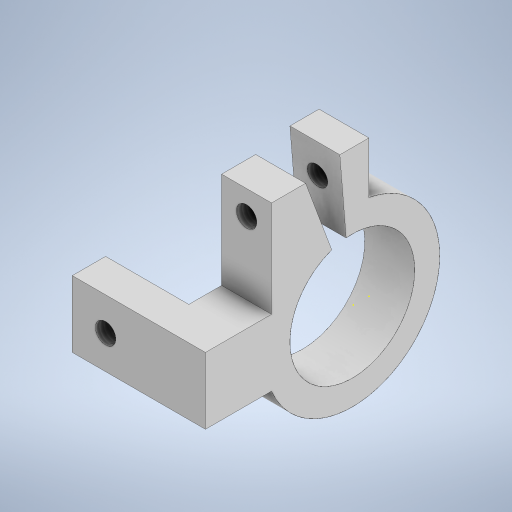
# Autodesk Inventor part: lensmount15mm
Saved by Autodesk Inventor 2023 (Build 270158000, 158)
## iProperties
Created: 2022-06-27
Part Number: lensmount15mm
Material: Generisch
Document SubType Name: Modeling
Designer: Tim Stechel
Density: 1 g/cm^3
Appearance: Vorgabe
Author: Tim Stechel
Autodesk Inventor part; units mm, degrees
ref_plane "YZ Plane" through (0, 0, 0) normal (1, 0, 0) x (0, 1, 0)
ref_plane "XZ Plane" through (0, 0, 0) normal (0, 1, 0) x (-1, 0, 0)
ref_plane "XY Plane" through (0, 0, 0) normal (0, 0, 1) x (1, 0, 0)
sketch "Skizze3" plane through (0, 0, 0) normal (0, 0, 1) x (1, 0, 0)
  line L0 (0, 0) -> (-6, 0)
  line L1 (-6, 0) -> (0, 0)
  line L2 (0, 7.5) -> (0, 10.5)
  line L3 (0, 10.5) -> (-6, 10.5)
  line L4 (-6, 10.5) -> (-6, 7.5)
  line L5 (-6, 7.5) -> (0, 7.5)
  dimension "d10" = 6
  dimension "d11" = 7.5
  dimension "d12" = 3
  dimension "d13" = 6
  constraints: 12 end point, 3 perpendicular, 1 collinear, 1 horizontal
  measures "d10" distance of L0.start L0.end
  measures "d11" distance of L0.start L2.start
  measures "d12" distance of L2.start L2.end
  measures "d13" distance of L2.end L3.end
revolve "Umdrehung2" add sketch "Skizze3" angle 335 about axis through (0, 0, 0) along (-1, 0, 0)
sketch "Skizze4" plane through (0, 7.5, 0) normal (1, 0, 0) x (0, 0, -1)
  circle A0 centre (0, -7.5) radius 7.5
  line L0 (-4.4375, 2.0162) -> (-3.1696, -0.7027) projected
  line L1 (-3.1696, -0.7027) -> (-6.9732, 7.4541)
  line L2 (-6.9732, 7.4541) -> (-5.6137, 8.088)
  line L3 (-5.6137, 8.088) -> (-2.474, -0.4198)
  line L4 (0, 0) -> (0, 3) projected
  line L5 (0, 0) -> (0, 9)
  line L6 (0, 9) -> (-1.5, 9)
  line L7 (-1.5, 9) -> (-0.7463, -0.0372)
  dimension "d15" = 9
  dimension "d17" = 1.5
  dimension "d18" = 9
  dimension "d19" = 1.5
  constraints: 12 end point, 2 point on circle, 1 centre point, 1 coincident, 1 collinear, 1 perpendicular, 1 vertical
  measures "d15" distance of L0.end L1.end
  measures "d17" distance of L1.end L2.end
  measures "d18" distance of L4.start L5.end
  measures "d19" distance of L5.end L6.end
extrude "Extrusion1" add sketch "Skizze4" against normal blind 6 contours A0 L7 L6 L5 L4 | L0 L1 L2 L3 A0
sketch "Skizze5" plane through (0, 7.0802, 2.474) normal (0, 0.3462167, -0.9381546) x (-1, 0, 0)
  point P0 (0, -7.4989)
sketch "Skizze6" plane through (-6, 10.5, 0) normal (-1, 0, 0) x (0, 0, 1)
  arc A0 (0, 0) -> (4.4375, -0.9838) centre (0, -10.5) ccw projected
  line L0 (0, -10.5) -> (17.6543, -10.5)
  line L1 (17.6543, -10.5) -> (17.6543, -14.5)
  line L2 (17.6543, -14.5) -> (17.6543, -10.5)
  line L3 (17.6543, -10.5) -> (17.6543, -6.5)
  line L4 (17.6543, -14.5) -> (9.7082, -14.5)
  line L5 (17.6543, -6.5) -> (9.7082, -6.5)
  point P0 (0, -10.5)
  dimension "d24" = 4
  dimension "d25" = 4
  constraints: 12 end point, 2 point on circle, 1 horizontal, 1 parallel
  measures "d24" distance of L0.end L1.end
  measures "d25" distance of L0.end L3.end
extrude "Extrusion2" add sketch "Skizze6" against normal blind 6
sketch "Skizze7" plane through (-6, 10.5, 0) normal (-1, 0, 0) x (0, 0, 1)
  line L0 (0, 6) -> (0, 0) projected
  line L1 (0, 6) -> (-2, 6)
  line L2 (-2, 6) -> (-2, -0.1922)
  arc A0 (0, 0) -> (9.7082, -14.5) centre (0, -10.5) ccw projected
  line L3 (4.4375, -0.9838) -> (6.9732, 4.4541) projected
  line L4 (6.9732, 4.4541) -> (5.6137, 5.088) projected
  line L5 (5.6137, 5.088) -> (9.6921, 3.1862)
  line L6 (9.6921, 3.1862) -> (6.9732, -2.6445)
  line L7 (9.6921, 3.1862) -> (6.9732, -2.6445)
  line L8 (9.6921, 3.1862) -> (6.9714, -2.6483)
  arc A1 (9.7082, -6.5) -> (4.4375, -0.9838) centre (0, -10.5) ccw projected
  arc A2 (9.7082, -6.5) -> (4.4375, -0.9838) centre (0, -10.5) ccw projected
  line L9 (9.7082, 5.088) -> (9.7082, -6.5)
  line L10 (9.7082, -6.5) -> (9.7082, 5.088)
  line L11 (9.7082, 5.088) -> (5.6137, 5.088)
  point P0 (0, -10.5)
  point P1 (6.9732, -2.6445)
  dimension "d28" = 2
  dimension "d30" = 4.5
  constraints: 18 end point, 3 perpendicular, 2 collinear, 2 point on circle, 1 horizontal, 1 point on line, 1 vertical
  measures "d28" distance of L0.start L1.end
  measures "d30" distance of L4.end L5.end
extrude "Extrusion3" add sketch "Skizze7" against normal blind 6
sketch "Skizze8" plane through (-6, -4, 17.6543) normal (-1, 0, 0) x (0, 0, 1)
  line L0 (0, 0) -> (-7.9461, 0) projected
  line L1 (-7.9461, 8) -> (0, 8) projected
  line L2 (0, 0) -> (-4, 0)
  line L3 (-4, 0) -> (-4, 8)
  line L4 (-4, 8) -> (0, 8)
  line L5 (0, 8) -> (0, 0)
  point P0 (-17.6543, 4)
  point P1 (-4, 0)
  dimension "d33" = 4
  constraints: 8 end point, 2 parallel, 1 horizontal, 1 perpendicular, 1 point on line
  measures "d33" distance of L3.end L4.end
extrude "Extrusion4" add sketch "Skizze8" along normal blind 10
sketch "Skizze9" plane through (-6, -4, 13.6543) normal (0, 0, -1) x (-1, 0, 0)
  line L0 (10, 8) -> (10, 0) projected
  line L1 (10, 4) -> (6, 4)
  circle A0 centre (6, 4) radius 1.5
  point P0 (-6, 4)
  dimension "d36" = 4
  dimension "d37" = 3
  constraints: 2 end point, 1 centre point, 1 coincident, 1 horizontal, 1 midpoint
  measures "d36" distance of L1.start L1.end
  measures "d37" diameter of A0
hole "Bohrung1" at (-12, 0, 13.6543) direction (0, 0, 1) diameter 2.459 end through all thread size "M3x0.5" class "6H" standard "ISO Metric profile"
sketch "Skizze10" plane through (-6, 10.3078, -2) normal (0, 0, -1) x (-1, 0, 0)
  point P0 (-6, -10.3078)
sketch "Skizze11" plane through (-6, 10.3078, -2) normal (0, 0, -1) x (-1, 0, 0)
  line L0 (0, 3.3785) -> (-6, 3.3785) projected
  line L1 (0, 3.3785) -> (-3, 3.3785)
  line L2 (-3, 3.3785) -> (-3, 2.3785)
  point P0 (-6, -10.3078)
  dimension "d46" = 3
  dimension "d47" = 1
  constraints: 4 end point, 1 midpoint, 1 perpendicular
  measures "d46" distance of L0.start L1.end
  measures "d47" distance of L1.end L2.end
hole "Bohrung3" at (-3, 12.6862, -2) direction (0, 0, 1) diameter 2.459 end through all thread size "M3x0.5" class "6H" standard "ISO Metric profile"
